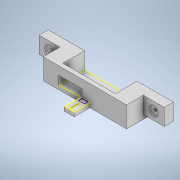
# Autodesk Inventor part: blah
Saved by Autodesk Inventor 2020 (Build 240168000, 168)
## iProperties
Created: 2019-11-12
Part Number: blah
Material: Generic
Document SubType Name: Modeling
Designer: bzs3334
Density: 1 g/cm^3
Appearance: Default
Author: bzs3334
Autodesk Inventor part; units mm, degrees
ref_plane "YZ Plane" through (0, 0, 0) normal (1, 0, 0) x (0, 1, 0)
ref_plane "XZ Plane" through (0, 0, 0) normal (0, 1, 0) x (-1, 0, 0)
ref_plane "XY Plane" through (0, 0, 0) normal (0, 0, 1) x (1, 0, 0)
sketch "Sketch1" plane through (0, 0, 0) normal (0, 1, 0) x (-1, 0, 0)
  line L0 (50, -15.5) -> (-50, -15.5)
  line L1 (-50, -15.5) -> (-50, 15.5)
  line L2 (-50, 15.5) -> (50, 15.5)
  line L3 (50, 15.5) -> (50, -15.5)
  line L4 (31.5, -15.5) -> (-31.5, -15.5)
  line L5 (-31.5, -15.5) -> (-31.5, 10.5)
  line L6 (-31.5, 10.5) -> (31.5, 10.5)
  line L7 (31.5, 10.5) -> (31.5, -15.5)
  line L8 (50, -15.5) -> (75, -15.5)
  line L9 (75, -15.5) -> (75, -4.5)
  line L10 (75, -4.5) -> (50, -4.5)
  line L11 (50, -4.5) -> (50, -15.5)
  line L12 (0, 0) -> (0, -15.5)
  line L13 (-50, -15.5) -> (-75, -15.5)
  line L14 (-75, -15.5) -> (-75, -4.5)
  line L15 (-75, -4.5) -> (-50, -4.5)
  point P0 (-50, -4.5)
  point P1 (-31.5, -15.5)
  dimension "d0" = 100
  dimension "d1" = 50
  dimension "d2" = 31
  dimension "d3" = 15.5
  dimension "d4" = 26
  dimension "d5" = 63
  dimension "d6" = 31.5
  dimension "d7" = 11
  dimension "d8" = 25
  constraints: 32 end point, 6 parallel, 3 horizontal, 3 perpendicular, 3 symmetric about line, 1 midpoint, 1 point on line
  measures "d0" distance of L0.start L0.end
  measures "d1" distance from line of L3 L12.start
  measures "d2" distance of L2.end L0.start
  measures "d3" distance from line of L2 L12.start
  measures "d4" distance of L6.end L4.start
  measures "d5" distance of L5.end L6.end
  measures "d6" distance from line of L5 L12.start
  measures "d7" distance of L8.end L9.end
  measures "d8" distance of L9.end L10.end
extrude "Extrusion1" add sketch "Sketch1" along normal blind 20 contours L0 L7 L6 L5 L1 L2 L3 | L3 L10 L9 L8 | L13 L14 L15 L1
sketch "Sketch2" plane through (-75, 0, -4.5) normal (0, 0, 1) x (1, 0, 0)
  line L0 (0, 0) -> (25, 0) projected
  line L1 (25, 0) -> (25, 20) projected
  line L2 (0, 20) -> (25, 20) projected
  line L3 (0, 0) -> (0, 20) projected
  circle A0 centre (12.5, 10) radius 1.75
  circle A1 centre (12.5, 10) radius 5.75
  point P0 (75, 0)
  dimension "d11" = 3.5
  dimension "d12" = 11.5
  constraints: 2 centre point, 1 coincident
  measures "d11" diameter of A0
  measures "d12" diameter of A1
extrude "Extrusion2" cut sketch "Sketch2" against normal through all contours A0
extrude "Extrusion3" cut sketch "Sketch2" against normal blind 2 contours A1
mirror "Mirror1" about plane through (0, 0, 0) normal (1, 0, 0) of "Extrusion3", "Extrusion2"
sketch "Sketch4" plane through (0, 0, 0) normal (0, -1, 0) x (1, 0, 0)
  line L0 (-31.5, -15.5) -> (-75, -15.5) projected
  line L1 (-31.5, 10.5) -> (-31.5, -15.5) projected
  line L2 (31.5, 10.5) -> (-31.5, 10.5) projected
  line L3 (31.5, -15.5) -> (31.5, 10.5) projected
  line L4 (75, -15.5) -> (31.5, -15.5) projected
  line L5 (75, -4.5) -> (75, -15.5) projected
  line L6 (50, -4.5) -> (75, -4.5) projected
  line L7 (50, 15.5) -> (50, -4.5) projected
  line L8 (-50, 15.5) -> (50, 15.5) projected
  line L9 (-50, -4.5) -> (-50, 15.5) projected
  line L10 (-75, -4.5) -> (-50, -4.5) projected
  line L11 (-75, -15.5) -> (-75, -4.5) projected
  line L12 (75, -15.5) -> (31.5, -15.5) projected
  line L13 (50, -15.5) -> (-50, -15.5)
  line L14 (-50, -15.5) -> (-50, 34.5)
  line L15 (-50, 34.5) -> (50, 34.5)
  line L16 (50, 34.5) -> (50, -15.5)
  point P0 (0, 0)
  dimension "d22" = 100
  dimension "d23" = 50
  constraints: 8 end point, 2 parallel, 1 horizontal, 1 perpendicular, 1 point on line
  measures "d22" distance of L14.end L15.end
  measures "d23" distance of L13.end L14.end
extrude "Extrusion5" add sketch "Sketch4" along normal blind 5 contours L0 L14 L9 L8 L7 L16 L4 L3 L2 L1 | L1 L2 L3 L13 | L14 L15 L16 L8
sketch "Sketch5" plane through (31.5, 20, 10.5) normal (0, 0, -1) x (-1, 0, 0)
  line L0 (63, -20) -> (0, -20) projected
  line L1 (63, -20) -> (35, -20)
  line L2 (35, -20) -> (35, -10)
  line L3 (35, -10) -> (63, -10)
  line L4 (63, -10) -> (63, -20)
  point P0 (31.5, -20)
  dimension "d26" = 28
  dimension "d27" = 10
  constraints: 8 end point, 2 parallel, 1 horizontal, 1 perpendicular
  measures "d26" distance of L2.end L3.end
  measures "d27" distance of L1.end L2.end
extrude "Extrusion6" cut sketch "Sketch5" against normal blind 57
sketch "Sketch6" plane through (0, 0, 0) normal (0, 1, 0) x (1, 0, 0)
  line L0 (-50, -15.5) -> (-31.5, -15.5) projected
  line L1 (-50, -34.5) -> (-50, -15.5) projected
  line L2 (50, -34.5) -> (-50, -34.5) projected
  line L3 (50, -15.5) -> (50, -34.5) projected
  line L4 (-3.5, -15.5) -> (50, -15.5) projected
  line L5 (-3.5, -10.5) -> (-3.5, -15.5) projected
  line L6 (31.5, -10.5) -> (-3.5, -10.5) projected
  line L7 (31.5, 15.5) -> (31.5, -10.5) projected
  line L8 (-31.5, 15.5) -> (31.5, 15.5) projected
  line L9 (-31.5, 15.5) -> (-31.5, -15.5) projected
  line L10 (-0.0641, -15.5) -> (-0.0641, -32.5)
  line L11 (-0.0641, -32.5) -> (-0.0641, -22.5) construction
  line L12 (0.7628, -32.5) -> (0.7628, -22.5)
  line L13 (-0.891, -22.5) -> (-0.891, -32.5)
  arc A0 (-0.891, -32.5) -> (0.7628, -32.5) centre (-0.0641, -32.5) ccw
  arc A1 (0.7628, -22.5) -> (-0.891, -22.5) centre (-0.0641, -22.5) ccw
  point P0 (0, 0)
  point P1 (-0.0641, -27.5)
  dimension "d36" = 10
  dimension "d37" = 2
  constraints: 10 end point, 4 point on circle, 4 tangent, 2 centre point, 2 point on line, 1 midpoint, 1 parallel, 1 perpendicular, 1 vertical
  measures "d36" distance of L12.start L12.end
  measures "d37" distance from line of L2 L10.end
extrude "Extrusion7" cut sketch "Sketch6" against normal blind 2 contours A1 L12 A0 L13
sketch "Sketch7" plane through (0, 0, 0) normal (0, 1, 0) x (1, 0, 0)
  line L0 (-3.5, -10.5) -> (-3.5, -15.5) projected
  arc A0 (-0.891, -32.5) -> (0.7628, -32.5) centre (-0.0641, -32.5) ccw projected
  line L1 (-0.891, -32.5) -> (-0.891, -22.5) projected
  arc A1 (0.7628, -22.5) -> (-0.891, -22.5) centre (-0.0641, -22.5) ccw projected
  line L2 (0.7628, -22.5) -> (0.7628, -32.5) projected
  line L3 (-50, -15.5) -> (-31.5, -15.5) projected
  line L4 (-50, -34.5) -> (-50, -15.5) projected
  line L5 (50, -34.5) -> (-50, -34.5) projected
  line L6 (50, -15.5) -> (50, -34.5) projected
  line L7 (-3.5, -15.5) -> (50, -15.5) projected
  line L8 (-3.5, -10.5) -> (-3.5, -15.5) projected
  line L9 (31.5, -10.5) -> (-3.5, -10.5) projected
  line L10 (31.5, 15.5) -> (31.5, -10.5) projected
  line L11 (-31.5, 15.5) -> (31.5, 15.5) projected
  line L12 (-31.5, 15.5) -> (-31.5, -15.5) projected
  line L13 (-3.5, -15.5) -> (50, -15.5) projected
  line L14 (50, -34.5) -> (-50, -34.5) projected
  line L15 (-3.5, -15.5) -> (-50, -15.5)
  line L16 (-50, -15.5) -> (-50, -34.5)
  line L17 (-50, -34.5) -> (-3.5, -34.5)
  line L18 (-3.5, -34.5) -> (-3.5, -15.5)
  line L19 (-50, -15.5) -> (50, -15.5) projected
  line L20 (-5.891, -34.5) -> (-50, -34.5)
  line L21 (-50, -34.5) -> (-50, -15.5)
  line L22 (-50, -15.5) -> (-5.891, -15.5)
  line L23 (-5.891, -15.5) -> (-5.891, -34.5)
  point P0 (0, 0)
  point P1 (-5.891, -34.5)
  point P2 (-5.891, -15.5)
  dimension "d32" = 5
  constraints: 16 end point, 4 parallel, 2 horizontal, 2 perpendicular, 1 point on line
  measures "d32" distance between parallel lines of L23 L1
extrude "Extrusion8" cut sketch "Sketch7" against normal blind 24.25 contours L23 L5 L4 L3 L15
mirror "Mirror2" about plane through (0, 0, 0) normal (1, 0, 0) of "Extrusion8"
sketch "Sketch10" plane through (0, 0, 0) normal (0, 1, 0) x (1, 0, 0)
  line L0 (-3.5, -10.5) -> (-3.5, -15.5) projected
  arc A0 (0.7628, -22.5) -> (-0.891, -22.5) centre (-0.0641, -22.5) ccw projected
  line L1 (0.7628, -22.5) -> (0.7628, -32.5) projected
  arc A1 (-0.891, -32.5) -> (0.7628, -32.5) centre (-0.0641, -32.5) ccw projected
  line L2 (-0.891, -32.5) -> (-0.891, -22.5) projected
  line L3 (5.891, -34.5) -> (5.891, -15.5) projected
  line L4 (-3.5, -15.5) -> (5.891, -15.5) projected
  line L5 (-3.5, -10.5) -> (-3.5, -15.5) projected
  line L6 (31.5, -10.5) -> (-3.5, -10.5) projected
  line L7 (31.5, 15.5) -> (31.5, -10.5) projected
  line L8 (-31.5, 15.5) -> (31.5, 15.5) projected
  line L9 (-31.5, 15.5) -> (-31.5, -15.5) projected
  line L10 (-31.5, -15.5) -> (-5.891, -15.5) projected
  line L11 (-5.891, -15.5) -> (-5.891, -34.5) projected
  line L12 (5.891, -34.5) -> (-5.891, -34.5) projected
  line L13 (-3.5, -15.5) -> (3.4148, -15.5)
  line L14 (3.4148, -15.5) -> (3.4148, -19.7081)
  line L15 (3.4148, -19.7081) -> (-3.5, -19.7081)
  line L16 (-3.5, -19.7081) -> (-3.5, -15.5)
  point P0 (0, 0)
  constraints: 8 end point, 2 parallel, 1 horizontal, 1 perpendicular
equation "\"d1\" = 0.5 * d0"
equation "\"d3\" = 0.5 * d2"
equation "\"d6\" = 0.5 * d5"
body "Solid1"
